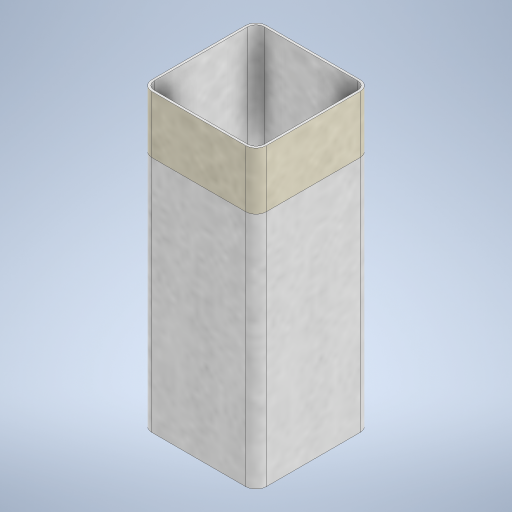
# Autodesk Inventor part: Fiberglass_isolation
Saved by Autodesk Inventor 2023 (Build 270158000, 158)
## iProperties
Created: 2022-09-23
Part Number: Fiberglass_isolation
Material: Стекловолоконная обертывающая изоляция
Document SubType Name: Modeling
Designer: Makar
Density: 0.0025 g/cm^3
Appearance: Полотно — белое
Mass: 0.0609953 g
Surface Area: 491.745 cm^2
Volume: 24.3981 cm^3
Author: Makar
Autodesk Inventor part; units mm, degrees
ref_plane "YZ Plane" through (0, 0, 0) normal (1, 0, 0) x (0, 1, 0)
ref_plane "XZ Plane" through (0, 0, 0) normal (0, 1, 0) x (-1, 0, 0)
sketch "Эскиз1" plane through (0, 0, 0) normal (0, 1, 0) x (-1, 0, 0)
  line L0 (-25, -20.5) -> (-25, 20.5)
  line L1 (-20.5, 25) -> (20.5, 25)
  line L2 (25, 20.5) -> (25, -20.5)
  line L3 (20.5, -25) -> (-20.5, -25)
  arc A0 (-25, -20.5) -> (-20.5, -25) centre (-20.5, -20.5) ccw
  arc A1 (-20.5, 25) -> (-25, 20.5) centre (-20.5, 20.5) ccw
  arc A2 (25, 20.5) -> (20.5, 25) centre (20.5, 20.5) ccw
  arc A3 (20.5, -25) -> (25, -20.5) centre (20.5, -20.5) ccw
  arc A4 (-20.5, 22) -> (-22, 20.5) centre (-20.5, 20.5) ccw
  line L4 (-20.5, 22) -> (20.5, 22)
  arc A5 (22, 20.5) -> (20.5, 22) centre (20.5, 20.5) ccw
  line L5 (22, 20.5) -> (22, -20.5)
  arc A6 (20.5, -22) -> (22, -20.5) centre (20.5, -20.5) ccw
  line L6 (20.5, -22) -> (-20.5, -22)
  arc A7 (-22, -20.5) -> (-20.5, -22) centre (-20.5, -20.5) ccw
  line L7 (-22, -20.5) -> (-22, 20.5)
  line L8 (0, 36.3048) -> (0, -36.3048) construction
  line L9 (-36.3048, 0) -> (36.3048, 0) construction
  arc A8 (20.5, -26) -> (26, -20.5) centre (20.5, -20.5) ccw
  line L10 (20.5, -26) -> (-20.5, -26)
  arc A9 (-26, -20.5) -> (-20.5, -26) centre (-20.5, -20.5) ccw
  line L11 (-26, -20.5) -> (-26, 20.5)
  arc A10 (-20.5, 26) -> (-26, 20.5) centre (-20.5, 20.5) ccw
  line L12 (-20.5, 26) -> (20.5, 26)
  arc A11 (26, 20.5) -> (20.5, 26) centre (20.5, 20.5) ccw
  line L13 (26, 20.5) -> (26, -20.5)
  arc A12 (20.5, -24) -> (24, -20.5) centre (20.5, -20.5) ccw
  line L14 (20.5, -24) -> (-20.5, -24)
  arc A13 (-24, -20.5) -> (-20.5, -24) centre (-20.5, -20.5) ccw
  line L15 (-24, -20.5) -> (-24, 20.5)
  arc A14 (-20.5, 24) -> (-24, 20.5) centre (-20.5, 20.5) ccw
  line L16 (-20.5, 24) -> (20.5, 24)
  arc A15 (24, 20.5) -> (20.5, 24) centre (20.5, 20.5) ccw
  line L17 (24, 20.5) -> (24, -20.5)
  point P0 (0, 0)
  dimension "d0" = 4.5
  dimension "d1" = 50
  dimension "d2" = 50
  dimension "d3" = 3
  dimension "d4" = 25
  dimension "d5" = 25
  dimension "d10" = 1
  dimension "d13" = 1
  constraints: 36 end point, 32 point on circle, 16 centre point, 8 parallel, 8 tangent, 4 perpendicular, 3 equal radius, 21 other
  measures "d0" radius of A0
  measures "d1" distance between parallel lines of L1 L3
  measures "d2" distance between parallel lines of L0 L2
  measures "d3" distance between parallel lines of L2 L5
  measures "d4" distance between parallel lines of L1 L9
  measures "d5" distance between parallel lines of L8 L2
  measures "d10" distance between parallel lines of L2 L13
  measures "d13" distance between parallel lines of L2 L17
extrude "Выдавливание1" add sketch "Эскиз1" along normal blind 129 contours L0 A1 L1 A2 L2 A3 L3 A0
ref_plane "РабПлоскость1" through (0, 104, 0) normal (0, 1, 0) x (1, 0, 0)
split_face "Разделение1"
equation "\"d0\" = d6"
equation "\"d1\" = d7"
equation "\"d2\" = d8"
equation "\"d3\" = d9"
equation "\"d4\" = 0.5 * d1"
equation "\"d5\" = 0.5 * d2"
equation "\"d6\" = 1.5 * d9"
equation "\"d7\" = 50"
equation "\"d8\" = 50"
equation "\"d9\" = 3"
